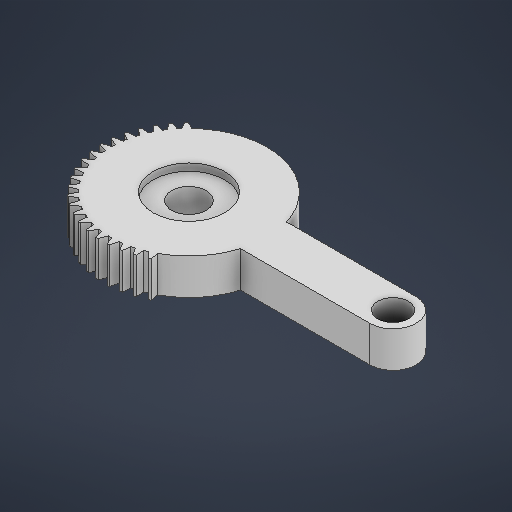
# Autodesk Inventor part: innerGear
Saved by Autodesk Inventor 2026.2 (Build 302298000, 298)
## iProperties
Created: 2026-04-07
Part Number: innerGear
Material: Generic
Document SubType Name: Modeling
Designer: Brian Wang
Density: 1 g/cm^3
Appearance: Default
Author: Brian Wang
Autodesk Inventor part; units mm, degrees
ref_plane "YZ Plane" through (0, 0, 0) normal (1, 0, 0) x (0, 1, 0)
ref_plane "XZ Plane" through (0, 0, 0) normal (0, 1, 0) x (-1, 0, 0)
ref_plane "XY Plane" through (0, 0, 0) normal (0, 0, 1) x (1, 0, 0)
sketch "Sketch1" plane through (0, 0, 0) normal (0, 1, 0) x (-1, 0, 0)
  circle A0 centre (0, 0) radius 11
  line L0 (0, 0) -> (21.5969, 0.9429) construction
  line L1 (0, 0) -> (22.384, -0.9773) construction
  line L2 (0, 0) -> (25.2479, 0) construction
  line L3 (10.9895, 0.4798) -> (12.0415, 0.1582)
  line L4 (10.9895, 0.4798) -> (12.0895, 0.4798) construction
  line L5 (10.9895, -0.4798) -> (12.0415, -0.1582)
  line L6 (12.0415, -0.1582) -> (12.0415, 0.1582)
  line L7 (10.9561, 0.9815) -> (11.9561, 1.4397)
  line L8 (11.9561, 1.4397) -> (11.9142, 1.7533)
  line L9 (10.8289, 1.9326) -> (11.9142, 1.7533)
  line L10 (10.7293, 2.4254) -> (11.6597, 3.0122)
  line L11 (11.6597, 3.0122) -> (11.5765, 3.3175)
  line L12 (10.4771, 3.3513) -> (11.5765, 3.3175)
  line L13 (10.313, 3.8266) -> (11.1574, 4.5315)
  line L14 (11.1574, 4.5315) -> (11.0345, 4.8231)
  line L15 (9.9402, 4.7109) -> (11.0345, 4.8231)
  line L16 (9.7146, 5.1602) -> (10.4581, 5.9708)
  line L17 (10.4581, 5.9708) -> (10.2976, 6.2435)
  line L18 (9.2279, 5.9872) -> (10.2976, 6.2435)
  line L19 (8.9446, 6.4026) -> (9.5741, 7.3047)
  line L20 (9.5741, 7.3047) -> (9.3789, 7.5537)
  line L21 (8.3526, 7.1578) -> (9.3789, 7.5537)
  line L22 (8.0168, 7.532) -> (8.521, 8.5096)
  line L23 (8.521, 8.5096) -> (8.2945, 8.7306)
  line L24 (7.3298, 8.2021) -> (8.2945, 8.7306)
  line L25 (6.9474, 8.5284) -> (7.3176, 9.5643)
  line L26 (7.3176, 9.5643) -> (7.0638, 9.7532)
  line L27 (6.1776, 9.1015) -> (7.0638, 9.7532)
  line L28 (5.7553, 9.3743) -> (5.9849, 10.45)
  line L29 (5.9849, 10.45) -> (5.7083, 10.6037)
  line L30 (4.9164, 9.8402) -> (5.7083, 10.6037)
  line L31 (4.4616, 10.0546) -> (4.5465, 11.1513)
  line L32 (4.5465, 11.1513) -> (4.252, 11.2669)
  line L33 (3.5683, 10.4052) -> (4.252, 11.2669)
  line L34 (3.0891, 10.5573) -> (3.0279, 11.6556)
  line L35 (3.0279, 11.6556) -> (2.7206, 11.7312)
  line L36 (2.1572, 10.7864) -> (2.7206, 11.7312)
  line L37 (1.6621, 10.8737) -> (1.4558, 11.9542)
  line L38 (1.4558, 11.9542) -> (1.1412, 11.9883)
  line L39 (0.708, 10.9772) -> (1.1412, 11.9883)
  line L40 (0.2057, 10.9981) -> (-0.142, 12.0417)
  line L41 (-0.142, 12.0417) -> (-0.4584, 12.0338)
  line L42 (-0.7536, 10.9742) -> (-0.4584, 12.0338)
  line L43 (-1.2543, 10.9283) -> (-1.7373, 11.9165)
  line L44 (-1.7373, 11.9165) -> (-2.0498, 11.8668)
  line L45 (-2.202, 10.7773) -> (-2.0498, 11.8668)
  line L46 (-2.6922, 10.6655) -> (-3.302, 11.581)
  line L47 (-3.302, 11.581) -> (-3.6051, 11.4902)
  line L48 (-3.6115, 10.3902) -> (-3.6051, 11.4902)
  line L49 (-4.0825, 10.2144) -> (-4.8083, 11.0409)
  line L50 (-4.8083, 11.0409) -> (-5.0967, 10.9108)
  line L51 (-4.9572, 9.8197) -> (-5.0967, 10.9108)
  line L52 (-5.4007, 9.5829) -> (-6.2297, 10.3059)
  line L53 (-6.2297, 10.3059) -> (-6.4983, 10.1387)
  line L54 (-6.2154, 9.0757) -> (-6.4983, 10.1387)
  line L55 (-6.6236, 8.7822) -> (-7.5411, 9.389)
  line L56 (-7.5411, 9.389) -> (-7.7852, 9.1876)
  line L57 (-7.3638, 8.1715) -> (-7.7852, 9.1876)
  line L58 (-7.7295, 7.8265) -> (-8.7194, 8.3062)
  line L59 (-8.7194, 8.3062) -> (-8.9346, 8.0743)
  line L60 (-8.3823, 7.1231) -> (-8.9346, 8.0743)
  line L61 (-8.699, 6.7326) -> (-9.7437, 7.0768)
  line L62 (-9.7437, 7.0768) -> (-9.9263, 6.8184)
  line L63 (-9.2527, 5.9488) -> (-9.9263, 6.8184)
  line L64 (-9.5148, 5.5198) -> (-10.596, 5.7225)
  line L65 (-10.596, 5.7225) -> (-10.7427, 5.4421)
  line L66 (-9.9597, 4.6695) -> (-10.7427, 5.4421)
  line L67 (-10.1627, 4.2095) -> (-11.2612, 4.2671)
  line L68 (-11.2612, 4.2671) -> (-11.3694, 3.9698)
  line L69 (-10.4909, 3.3078) -> (-11.3694, 3.9698)
  line L70 (-4.2364, 41.6401) -> (-4.9873, 42.4439)
  line L71 (-4.2364, 41.6401) -> (-4.7195, 42.6284) construction
  line L72 (-5.0986, 41.2187) -> (-5.2716, 42.305)
  line L73 (-5.2716, 42.305) -> (-4.9873, 42.4439)
  line L74 (-3.7882, 41.8237) -> (-3.8157, 42.9233)
  line L75 (-3.8157, 42.9233) -> (-3.5155, 43.0234)
  line L76 (-2.8778, 42.1271) -> (-3.5155, 43.0234)
  line L77 (-2.4093, 42.2496) -> (-2.2907, 43.3432)
  line L78 (-2.2907, 43.3432) -> (-1.9799, 43.4025)
  line L79 (-1.4667, 42.4296) -> (-1.9799, 43.4025)
  line L80 (-0.9861, 42.4889) -> (-0.7236, 43.5571)
  line L81 (-0.7236, 43.5571) -> (-0.4077, 43.5747)
  line L82 (-0.028, 42.5423) -> (-0.4077, 43.5747)
  line L83 (0.4561, 42.5374) -> (0.858, 43.5614)
  line L84 (0.858, 43.5614) -> (1.1734, 43.537)
  line L85 (1.4129, 42.4634) -> (1.1734, 43.537)
  line L86 (1.892, 42.3943) -> (2.4261, 43.3559)
  line L87 (2.4261, 43.3559) -> (2.7355, 43.2899)
  line L88 (2.8305, 42.194) -> (2.7355, 43.2899)
  line L89 (3.2962, 42.0621) -> (3.953, 42.9444)
  line L90 (3.953, 42.9444) -> (4.251, 42.8379)
  line L91 (4.1998, 41.7391) -> (4.251, 42.8379)
  line L92 (4.6438, 41.5466) -> (5.4119, 42.3341)
  line L93 (5.4119, 42.3341) -> (5.6931, 42.1891)
  line L94 (5.4967, 41.1067) -> (5.6931, 42.1891)
  line L95 (5.9112, 40.8571) -> (6.7768, 41.5358)
  line L96 (6.7768, 41.5358) -> (7.0363, 41.3548)
  line L97 (6.6982, 40.308) -> (7.0363, 41.3548)
  line L98 (7.0759, 40.0057) -> (8.0239, 40.5636)
  line L99 (8.0239, 40.5636) -> (8.2571, 40.3498)
  line L100 (7.7831, 39.3571) -> (8.2571, 40.3498)
  line L101 (8.1173, 39.0074) -> (9.1309, 39.4347)
  line L102 (9.1309, 39.4347) -> (9.3337, 39.1919)
  line L103 (8.7324, 38.2708) -> (9.3337, 39.1919)
  line L104 (9.0172, 37.8799) -> (10.0785, 38.1691)
  line L105 (10.0785, 38.1691) -> (10.2473, 37.9015)
  line L106 (9.5291, 37.0683) -> (10.2473, 37.9015)
  line L107 (9.7596, 36.6432) -> (10.8499, 36.7891)
  line L108 (10.8499, 36.7891) -> (10.9817, 36.5014)
  line L109 (10.1594, 35.7708) -> (10.9817, 36.5014)
  line L110 (10.3315, 35.319) -> (11.4315, 35.319)
  line L111 (11.4315, 35.319) -> (11.524, 35.0164)
  line L112 (10.6121, 34.4013) -> (11.524, 35.0164)
  line L113 (10.7227, 33.9307) -> (11.813, 33.7849)
  line L114 (11.813, 33.7849) -> (11.8645, 33.4727)
  line L115 (10.8791, 32.9839) -> (11.8645, 33.4727)
  line L116 (10.9263, 32.5029) -> (11.9877, 32.2138)
  line L117 (11.9877, 32.2138) -> (11.9974, 31.8975)
  line L118 (10.9559, 31.5437) -> (11.9974, 31.8975)
  line L119 (10.9389, 31.0607) -> (11.9526, 30.6335)
  line L120 (11.9526, 30.6335) -> (11.9203, 30.3187)
  line L121 (10.841, 30.1061) -> (11.9203, 30.3187)
  line L122 (10.7602, 29.6297) -> (11.7083, 29.0719)
  line L123 (11.7083, 29.0719) -> (11.6345, 28.7642)
  line L124 (10.5366, 28.6965) -> (11.6345, 28.7642)
  line L125 (10.3934, 28.2352) -> (11.2591, 27.5565)
  line L126 (11.2591, 27.5565) -> (11.1452, 27.2613)
  line L127 (10.048, 27.3398) -> (11.1452, 27.2613)
  line L128 (9.8449, 26.9016) -> (10.613, 26.1142)
  line L129 (10.613, 26.1142) -> (10.461, 25.8367)
  line L130 (9.3839, 26.0599) -> (10.461, 25.8367)
  line L131 (9.1245, 25.6526) -> (9.7814, 24.7703)
  line L132 (9.7814, 24.7703) -> (9.5939, 24.5154)
  line L133 (8.5559, 24.8795) -> (9.5939, 24.5154)
  line L134 (8.2449, 24.5102) -> (8.779, 23.5485)
  line L135 (8.779, 23.5485) -> (8.5594, 23.3207)
  line L136 (7.5789, 23.8193) -> (8.5594, 23.3207)
  circle A1 centre (-28.2592, 31.6849) radius 2.125
  arc A2 (-28.2592, 34.8924) -> (-28.2592, 28.4774) centre (-28.2592, 31.6849) ccw
  line L137 (-28.2592, 34.8924) -> (-10.2739, 34.8924)
  line L138 (-28.2592, 28.4774) -> (-10.2623, 28.4774)
  line L139 (18.6565, 53.6502) -> (-47.4327, 53.6502)
  line L140 (18.6565, 53.6502) -> (84.7457, 53.6502) construction
  circle A3 centre (0.1033, 31.6831) radius 2.4
  arc A4 (-5.0986, 41.2187) -> (-10.2739, 34.8924) centre (0.1033, 31.6831) ccw
  arc A5 (-3.7882, 41.8237) -> (-4.2364, 41.6401) centre (0.1033, 31.6831) ccw
  arc A6 (-2.4093, 42.2496) -> (-2.8778, 42.1271) centre (0.1033, 31.6831) ccw
  arc A7 (-0.9861, 42.4889) -> (-1.4667, 42.4296) centre (0.1033, 31.6831) ccw
  arc A8 (0.4561, 42.5374) -> (-0.028, 42.5423) centre (0.1033, 31.6831) ccw
  arc A9 (1.892, 42.3943) -> (1.4129, 42.4634) centre (0.1033, 31.6831) ccw
  arc A10 (3.2962, 42.0621) -> (2.8305, 42.194) centre (0.1033, 31.6831) ccw
  arc A11 (4.6438, 41.5466) -> (4.1998, 41.7391) centre (0.1033, 31.6831) ccw
  arc A12 (5.9112, 40.8571) -> (5.4967, 41.1067) centre (0.1033, 31.6831) ccw
  arc A13 (7.0759, 40.0057) -> (6.6982, 40.308) centre (0.1033, 31.6831) ccw
  arc A14 (8.1173, 39.0074) -> (7.7831, 39.3571) centre (0.1033, 31.6831) ccw
  arc A15 (9.0172, 37.8799) -> (8.7324, 38.2708) centre (0.1033, 31.6831) ccw
  arc A16 (9.7596, 36.6432) -> (9.5291, 37.0683) centre (0.1033, 31.6831) ccw
  arc A17 (10.3315, 35.319) -> (10.1594, 35.7708) centre (0.1033, 31.6831) ccw
  arc A18 (10.7227, 33.9307) -> (10.6121, 34.4013) centre (0.1033, 31.6831) ccw
  arc A19 (10.9263, 32.5029) -> (10.8791, 32.9839) centre (0.1033, 31.6831) ccw
  arc A20 (10.9389, 31.0607) -> (10.9559, 31.5437) centre (0.1033, 31.6831) ccw
  arc A21 (10.7602, 29.6297) -> (10.841, 30.1061) centre (0.1033, 31.6831) ccw
  arc A22 (10.3934, 28.2352) -> (10.5366, 28.6965) centre (0.1033, 31.6831) ccw
  arc A23 (9.8449, 26.9016) -> (10.048, 27.3398) centre (0.1033, 31.6831) ccw
  arc A24 (9.1245, 25.6526) -> (9.3839, 26.0599) centre (0.1033, 31.6831) ccw
  arc A25 (-10.2623, 28.4774) -> (7.5789, 23.8193) centre (0.1033, 31.6831) ccw
  arc A26 (8.2449, 24.5102) -> (8.5559, 24.8795) centre (0.1033, 31.6831) ccw
  dimension "d0" = 22
  dimension "d1" = 2.5
  dimension "d2" = 2.5
  dimension "d3" = 1.1
  dimension "d4" = 17
  dimension "d5" = 0.3164
  dimension "d8" = 160
  dimension "d12" = 4.25
  dimension "d16" = 4.8
  dimension "d21" = 10.85
  constraints: 282 end point, 48 point on circle, 45 point on line, 26 centre point, 4 coincident, 4 horizontal, 2 equal length, 2 symmetric about line, 2 tangent, 1 parallel, 1 vertical, 172 other
  measures "d1" angle of L2 L0
  measures "d2" angle of L1 L2
  measures "d3" distance of L3.start L3.end
  measures "d4" angle of L3 L4
  measures "d5" distance of L5.end L6.end
  measures "d12" diameter of A1
  measures "d16" diameter of A3
  measures "d21" radius of A25
extrude "Extrusion1" add sketch "Sketch1" along normal blind 5 contours A5 L74 L75 L76 A6 L77 L78 L79 A7 L80 L81 L82 A8 L83 L84 L85 A9 L86 L87 L88 A10 L89 L90 L91 A11 L92 L93 L94 A12 L95 L96 L97 A13 L98 L99 L100 A14 L101 L102 L103 A15 L104 L105 L106 A16 L107 L108 L109 A17 L110 L111 L112 A18 L113 L114 L115 A19 L116 L117 L118 A20 L119 L120 L121 A21 L122 L123 L124 A22 L125 L126 L127 A23 L128 L129 L130 A24 L131 L132 L133 A26 L134 L135 L136 A25 L138 A2 L137 A4 L72 L73 L70
sketch "Sketch2" plane through (0, 5, 0) normal (0, 1, 0) x (1, 0, 0)
  circle A0 centre (-0.1033, -31.6831) radius 2.4 projected
  circle A1 centre (-0.1033, -31.6831) radius 4.9724
  point P0 (0, 0)
  constraints: 1 centre point, 1 coincident
extrude "Extrusion2" cut sketch "Sketch2" against normal blind 1
body "Solid1"
